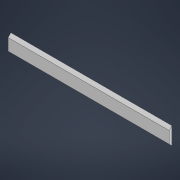
# Autodesk Inventor part: goalPanelBack
Saved by Autodesk Inventor 2021 (Build 250183000, 183)
## iProperties
Created: 2021-11-24
Part Number: goalPanelBack
Material: Generic
Document SubType Name: Modeling
Designer: jo_ki
Density: 1 g/cm^3
Appearance: Default
Author: jo_ki
Autodesk Inventor part; units mm, degrees
ref_plane "YZ Plane" through (0, 0, 0) normal (1, 0, 0) x (0, 1, 0)
ref_plane "XZ Plane" through (0, 0, 0) normal (0, 1, 0) x (-1, 0, 0)
ref_plane "XY Plane" through (0, 0, 0) normal (0, 0, 1) x (1, 0, 0)
derived "Mastersketch.ipt"
sketch "Sketch1" plane through (0, 0, 0) normal (1, 0, 0) x (0, 1, 0)
  line L0 (8.5, 2) -> (-8.5, 2)
  line L1 (8.5, 2) -> (12.5, -2)
  line L2 (12.5, -2) -> (-12.5, -2)
  line L3 (-12.5, -2) -> (-8.5, 2)
  line L4 (0, -2.8) -> (0, 2.8) projected
  line L5 (-17.5, 0) -> (17.5, 0) projected
  point P0 (0, 0)
  dimension "d0" = 45
  dimension "d2" = 45
  dimension "d3" = 4
  dimension "d5" = 25
  constraints: 8 end point, 1 horizontal, 1 parallel, 1 symmetric about line, 1 other
  measures "d0" angle of L4 L1
  measures "d2" angle of L4 L3
  measures "d3" distance between parallel lines of L0 L2
  measures "d5" distance of L2.end L1.end
derived "goalPanelSide.ipt"
extrude "Extrusion1" add sketch "Sketch1" along normal blind 232
equation "\"d0\" = goalCollector_angle"
equation "\"d2\" = goalCollectorRollback_angle"
equation "\"d3\" = goalPanel_thickness"
equation "\"d5\" = goalStructureBack_height"
equation "\"d6\" = goal_width + 2 * goalPanel_thickness"
equation "\"goalCollector_angle\" = 45deg"
equation "\"goalCollectorRollback_angle\" = 45deg"
equation "\"goalPanel_thickness\" = 4"
equation "\"goalStructureBack_height\" = 25"
equation "\"goal_width\" = 224"
body "Solid1"
